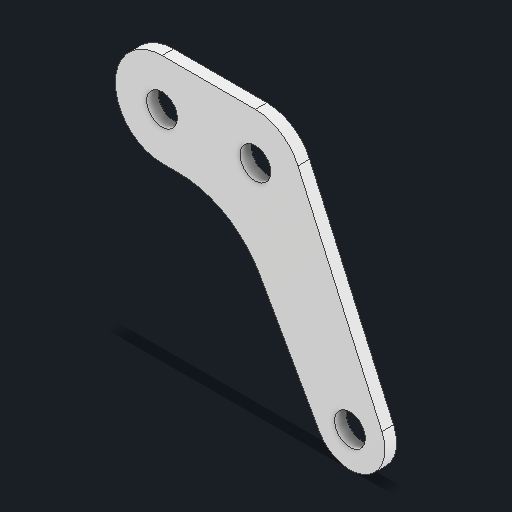
# Autodesk Inventor part: Clamp Gusset
Saved by Autodesk Inventor 2025.1 (Build 291241000, 241)
## iProperties
Created: 2024-11-12
Part Number: Clamp Gusset
Material: Acetal Resin, White
Document SubType Name: Modeling
Designer: avere
Density: 1.425 g/cm^3
Appearance: Smooth - White
Author: avere
Autodesk Inventor part; units mm, degrees
ref_plane "YZ Plane" through (0, 0, 0) normal (1, 0, 0) x (0, 1, 0)
ref_plane "XZ Plane" through (0, 0, 0) normal (0, 1, 0) x (-1, 0, 0)
ref_plane "XY Plane" through (0, 0, 0) normal (0, 0, 1) x (1, 0, 0)
sketch "Sketch1" plane through (0, 0, 0) normal (0, 0, 1) x (1, 0, 0)
  circle A0 centre (0, 0) radius 2.0955
  circle A1 centre (-12.7, 0) radius 2.0955
  arc A2 (-12.7, 6.35) -> (-12.7, -6.35) centre (-12.7, 0) ccw
  arc A3 (5.7981, 2.5893) -> (0, 6.35) centre (0, 0) ccw
  line L0 (0, 0) -> (32.8335, 0) construction
  line L1 (15.0623, -29.1748) -> (10.0742, -31.75)
  line L2 (-10.4687, -6.35) -> (-12.7, -6.35)
  arc A4 (8.7261, -27.2769) -> (17.2261, -23.001) centre (12.8775, -24.943) ccw
  line L3 (17.2261, -23.001) -> (5.7981, 2.5893)
  line L4 (0.6017, -12.8261) -> (8.7261, -27.2769)
  line L5 (-12.7, 6.35) -> (0, 6.35)
  arc A5 (0.6017, -12.8261) -> (-10.4687, -6.35) centre (-10.4687, -19.05) ccw
  circle A6 centre (12.8775, -24.943) radius 2.0955
  dimension "d0" = 4.191
  dimension "d1" = 32.8335
  dimension "d3" = 9.525
  dimension "d4" = 12.7
  dimension "d5" = 4.191
  constraints: 12 end point, 8 point on circle, 7 centre point, 7 tangent, 4 coincident, 2 horizontal, 1 other
  measures "d0" diameter of A0
  measures "d1" distance of L0.start L1.start
  measures "d3" diameter of A4
  measures "d4" radius of A5
  measures "d5" diameter of A6
extrude "Extrusion1" add sketch "Sketch1" along normal blind 1.5875
body "Solid1"
